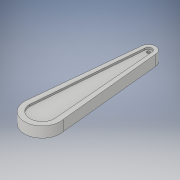
# Autodesk Inventor part: Delta_Arm
Saved by Autodesk Inventor 2019 (Build 230136000, 136)
## iProperties
Created: 2019-08-29
Part Number: Delta_Arm
Material: Generic
Document SubType Name: Modeling
Designer: Jorian Brusind
Density: 1 g/cm^3
Appearance: Default
Author: Jorian Brusind
Autodesk Inventor part; units mm, degrees
ref_plane "YZ Plane" through (0, 0, 0) normal (1, 0, 0) x (0, 1, 0)
ref_plane "XZ Plane" through (0, 0, 0) normal (0, 1, 0) x (-1, 0, 0)
ref_plane "XY Plane" through (0, 0, 0) normal (0, 0, 1) x (1, 0, 0)
sketch "Sketch1" plane through (0, 0, 0) normal (0, 1, 0) x (-1, 0, 0)
  circle A0 centre (0, 0) radius 25
  line L0 (0, 0) -> (0, -150)
  circle A1 centre (0, -150) radius 10
  line L1 (0, 0) -> (25, 0)
  line L2 (0, -150) -> (10, -150)
  line L3 (0, -150) -> (-10, -150)
  line L4 (0, 0) -> (-25, 0)
  line L5 (25, 0) -> (10, -150)
  line L6 (-25, 0) -> (-10, -150)
  dimension "d0" = 50
  dimension "d1" = 150
  dimension "d2" = 20
  constraints: 14 end point, 4 point on circle, 2 centre point, 2 coincident, 2 point on line, 1 horizontal, 1 parallel, 1 vertical
  measures "d0" diameter of A0
  measures "d1" distance of L0.start L0.end
  measures "d2" diameter of A1
extrude "Extrusion1" add sketch "Sketch1" along normal blind 15
sketch "Sketch2" plane through (0, 15, 0) normal (0, 1, 0) x (1, 0, 0)
  circle A0 centre (0, 0) radius 17.5
  arc A1 (10, 150) -> (-10, 150) centre (0, 150) ccw projected
  circle A2 centre (0, 150) radius 5
  line L0 (0, 0) -> (-17.5, 0)
  line L1 (0, 0) -> (17.5, 0)
  line L2 (0, 150) -> (-5, 150)
  line L3 (0, 150) -> (5, 150)
  line L4 (-17.5, 0) -> (-5, 150)
  line L5 (5, 150) -> (17.5, 0)
  dimension "d5" = 35
  dimension "d6" = 10
  constraints: 12 end point, 4 point on circle, 2 centre point, 2 coincident, 2 point on line, 1 horizontal, 1 parallel
  measures "d5" diameter of A0
  measures "d6" diameter of A2
extrude "Extrusion2" cut sketch "Sketch2" against normal blind 2.5 contours L0 L1 A0 | L4 A0 L5 L1 L0 | L4 A2 L5 A0 | L2 L3 A2 | A2 L3 L2
sketch "Sketch3" plane through (0, 12.5, 0) normal (0, 1, 0) x (1, 0, 0)
  arc A0 (5, 150) -> (-5, 150) centre (0, 150) ccw projected
  circle A1 centre (0, 150) radius 2.25
  point P0 (0, 0)
  dimension "d9" = 4.5
  constraints: 1 centre point, 1 coincident
  measures "d9" diameter of A1
extrude "Extrusion3" cut sketch "Sketch3" against normal blind 12.5
body "Solid1"
